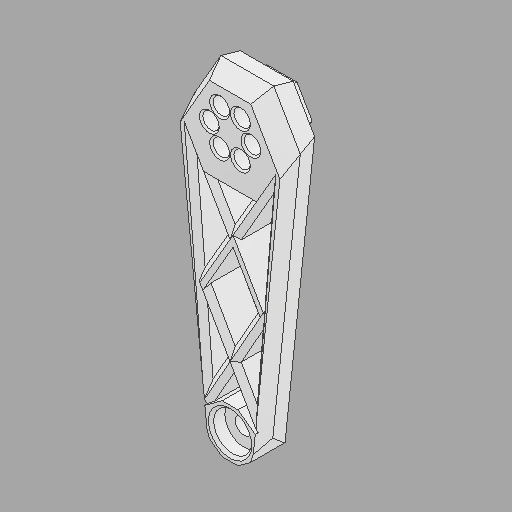
# Autodesk Inventor part: UPPER_LINKAGE_LH_V2
Saved by Autodesk Inventor 2025.2 (Build 292293000, 293)
## iProperties
Created: 2026-05-25
Part Number: UPPER_LINKAGE_LH_V2
Material: ABS Plastic
Document SubType Name: Modeling
Designer: Ben
Density: 1.06 g/cm^3
Appearance: Smooth - White
Mass: 110.874 g
Surface Area: 371.231 cm^2
Volume: 104.598 cm^3
Author: Ben
Autodesk Inventor part; units mm, degrees
ref_plane "YZ Plane" through (0, 0, 0) normal (1, 0, 0) x (0, 1, 0)
ref_plane "XZ Plane" through (0, 0, 0) normal (0, 1, 0) x (-1, 0, 0)
ref_plane "XY Plane" through (0, 0, 0) normal (0, 0, 1) x (1, 0, 0)
sketch "Sketch1" plane through (0, 0, 0) normal (0, 0, 1) x (1, 0, 0)
  circle A0 centre (0, 0) radius 26.5
  circle A1 centre (0, -150) radius 14
  line L0 (-26.407826, -2.208333) -> (-13.951304, -151.166667)
  line L1 (26.407826, -2.208333) -> (13.951304, -151.166667)
  line L2 (-42.83939, 0) -> (42.83939, 0)
  line L3 (30.599564, 0) -> (15.299782, 26.5)
  line L4 (15.299782, 26.5) -> (-15.299782, 26.5)
  line L5 (-15.299782, 26.5) -> (-30.599564, 0)
  line L6 (14.720471, -150) -> (11.909111, -158.652476)
  line L7 (11.909111, -158.652476) -> (4.548876, -164)
  line L8 (4.548876, -164) -> (-4.548876, -164)
  line L9 (-4.548876, -164) -> (-11.909111, -158.652476)
  line L10 (-11.909111, -158.652476) -> (-14.720471, -150)
  line L11 (30.599564, 0) -> (14.720471, -150)
  line L12 (-30.599564, 0) -> (-14.720471, -150)
  line L13 (30.599564, 0) -> (15.299782, -26.5)
  line L14 (15.299782, -26.5) -> (-15.299782, -26.5)
  line L15 (-30.599564, 0) -> (-15.299782, -26.5)
  line L16 (14.720471, -150) -> (11.909111, -141.347524)
  line L17 (11.909111, -141.347524) -> (4.548876, -136)
  line L18 (4.548876, -136) -> (-4.548876, -136)
  line L19 (-4.548876, -136) -> (-11.909111, -141.347524)
  line L20 (-11.909111, -141.347524) -> (-14.720471, -150)
  line L21 (22.949673, -13.25) -> (11.909111, -141.347524)
  line L22 (-11.909111, -141.347524) -> (-22.949673, -13.25)
  line L23 (22.341795, -20.302876) -> (-16.537733, -87.644193)
  line L24 (11.835681, -26.5) -> (-17.437654, -77.202903)
  line L25 (15.299782, -26.5) -> (-16.987693, -82.423548) construction
  line L26 (-15.299782, -26.5) -> (16.987693, -82.423548) construction
  line L27 (-22.341795, -20.302876) -> (16.537733, -87.644193)
  line L28 (17.437654, -77.202903) -> (-11.835681, -26.5)
  line L29 (17.437654, -77.202903) -> (-12.821294, -130.763976)
  line L30 (16.197037, -91.597102) -> (-11.909111, -141.347524)
  line L31 (-17.437654, -77.202903) -> (12.821294, -130.763976)
  line L32 (-16.197037, -91.597102) -> (11.909111, -141.347524)
  point P0 (-26.5, 0)
  point P1 (26.5, 0)
  point P2 (-22.949673, 13.25)
  point P3 (0, 26.5)
  point P4 (22.949673, 13.25)
  point P5 (13.314791, -154.326238)
  point P6 (-13.314791, -154.326238)
  point P7 (-8.228994, -161.326238)
  point P8 (0, -164)
  point P9 (8.228994, -161.326238)
  point P10 (-3.464102, -53)
  point P11 (0, -59)
  point P12 (3.464102, -53)
  point P13 (0, -47)
  point P14 (3.445641, -114.168224)
  point P15 (14.011179, -83.268074)
  point P16 (0, -108.069127)
  point P17 (-14.011179, -83.268074)
  point P18 (-3.445641, -114.168224)
  point P19 (0, -120.267321)
  dimension "d0" = 53
  dimension "d1" = 28
  dimension "d2" = 150
  dimension "d50" = 360
  dimension "d60" = 360
  dimension "d68" = 6
  dimension "d69" = 6
  dimension "d70" = 6
  dimension "d71" = 6
  constraints: 60 end point, 6 tangent, 5 parallel, 4 point on circle, 3 coincident, 3 point on line, 2 centre point, 2 collinear, 2 horizontal, 2 midpoint, 1 horizontal alignment, 1 vertical alignment, 40 other
  measures "d0" diameter of A0
  measures "d1" diameter of A1
  measures "d2" distance of A1.centre point (0, 0)
  measures "d68" distance between parallel lines of L24 L23
  measures "d69" distance between parallel lines of L27 L28
  measures "d70" distance between parallel lines of L32 L31
  measures "d71" distance between parallel lines of L30 L29
extrude "Extrusion1" add sketch "Sketch1" along normal blind 20 contours A0 L2 | L0 L15 L2 A0 | A0 L15 L0 | A0 L14 L15 | L22 L20 L0 L15 | L15 L14 L28 L24 L27 L22 | L2 L5 A0 | A0 L2 | L0 L20 L12 L15 | A0 L13 L14 | L5 L4 A0 | L2 L13 L1 A0 | A0 L3 L2 | L20 A1 L0 | L0 A1 L10 L20 | L21 L23 L28 L24 L14 L13 | A0 L1 L13 | L13 L1 L16 L21 | L31 L23 L22 | L24 L27 L23 L31 | L24 L28 L23 L27 | L4 L3 A0 | L11 L16 L1 L13 | A1 | L20 L19 A1 | L23 L31 L29 L32 L22 | L23 L28 L29 L27 | A1 L9 L10 | L6 A1 L1 L16 | L19 L18 A1 | L22 L29 L32 L30 | L1 A1 L16 | L21 L27 L29 | L31 L30 L32 L29 | L29 L27 L21 L30 L31 | A1 L8 L9 | L6 L7 A1 | L18 L17 A1 | L30 L31 L21 L32 | A1 L17 L16 | A1 L7 L8
sketch "Sketch2" plane through (0, 0, 20) normal (0, 0, 1) x (1, 0, 0)
  line L0 (0, -202.1) -> (0, 64.6)
  line L1 (-6, 10.392305) -> (0, 0) construction
  point P0 (6, 10.392305)
  point P1 (-6, -10.392305)
  point P2 (-12, 0)
  point P3 (12, 0)
  point P4 (6, -10.392305)
  dimension "d18" = 12
  dimension "d19" = 12
  dimension "d22" = 360
  constraints: 2 coincident, 2 end point, 1 symmetric about line, 8 other
  measures "d18" distance of point (6, 10.392) L1.start
  measures "d19" distance of L1.start L1.end
sketch "Sketch3" plane through (0, 0, 20) normal (0, 0, 1) x (1, 0, 0)
  arc A0 (-14.98591, -150.65) -> (14.98591, -150.65) centre (0, -150) ccw
  point P0 (0, 0)
  constraints: 1 coincident
hole "Hole2" at (0, -150, 20) direction (0, 0, -1) diameter 10 end through all counterbore diameter 22 counterbore depth 8
chamfer "Chamfer4" distance 1.5 angle 45 1 edges at (0, -139, 20)
chamfer "Chamfer5" distance 10 angle 30 1 edges at (22.9497, 13.25, 20) measured on face at (22.9497, 13.25, 19.5)
chamfer "Chamfer6" distance 10 angle 30 1 edges at (-3.3333, 26.5, 20) measured on face at (-3.3333, 26.5, 19.5)
chamfer "Chamfer7" distance 10 angle 30 1 edges at (-24.6163, 10.3632, 20) measured on face at (-24.6163, 10.3632, 19.5)
chamfer "Chamfer8" distance 10 angle 5 1 edges at (-22.1435, -79.8789, 20) measured on face at (-22.1435, -79.8789, 19.5)
chamfer "Chamfer9" distance 10 angle 5 1 edges at (22.1435, -79.8789, 20) measured on face at (22.1435, -79.8789, 19.5)
chamfer "Chamfer10" distance 3 angle 45 18 edges at (19.8897, -48.7529, 20) (12.9029, -36.6514, 20) (5.9178, -36.75, 20) (-5.9178, -36.75, 20) (-12.9029, -36.6514, 20) (-10.4509, -65.1015, 20) (-19.8897, -48.7529, 20) (7.0056, -71.134, 20) (-7.0056, -95.6686, 20) (-9.8213, -102.8827, 20) (-8.1335, -122.4661, 20) (-5.9546, -130.8074, 20) (5.9546, -130.8074, 20) (8.1335, -122.4661, 20) (14.5092, -111.1805, 20) (9.8213, -102.8827, 20) (7.0056, -95.6686, 20) (-14.5092, -111.1805, 20)
sketch "Sketch4" plane through (0, 0, 0) normal (0, 0, -1) x (-1, 0, 0)
  line L0 (-8.75, 15.155445) -> (-17.5, 0)
  line L1 (-17.5, 0) -> (-8.75, -15.155445)
  line L2 (-8.75, -15.155445) -> (8.75, -15.155445)
  line L3 (8.75, -15.155445) -> (17.5, 0)
  line L4 (17.5, 0) -> (8.75, 15.155445)
  line L5 (8.75, 15.155445) -> (-8.75, 15.155445)
  point P0 (0, 0)
  dimension "d91" = 17.5
  dimension "d94" = 360
  constraints: 12 end point, 3 parallel, 1 horizontal, 1 horizontal alignment, 7 other
  measures "d91" distance of point (0, 0) L0.end
extrude "Extrusion2" add sketch "Sketch4" along normal blind 10
hole "Hole3" at (-6, 10.392305, 20) at (6, 10.392305, 20) at (-6, -10.392305, 20) at (-12, 0, 20) at (12, 0, 20) at (6, -10.392305, 20) direction (0, 0, -1) diameter 4.5 end through all counterbore diameter 9.5 counterbore depth 15
chamfer "Chamfer11" distance 1 angle 45 6 edges at (-12, 4.75, 20) (-6, -5.6423, 20) (6, -5.6423, 20) (12, 4.75, 20) (6, 15.1423, 20) (-6, 15.1423, 20)
chamfer "Chamfer12" distance 2 distance2 10 6 edges at (0, 15.1554, 0) (13.125, 7.5777, 0) (13.125, -7.5777, 0) (0, -15.1554, 0) (-13.125, -7.5777, 0) (-13.125, 7.5777, 0) measured on face at (13.558, -7.8277, 0) measured on face at (0, 15.6554, 0) measured on face at (13.558, 7.8277, 0) measured on face at (-13.558, 7.8277, 0) measured on face at (0, -15.6554, 0) measured on face at (-13.558, -7.8277, 0)
chamfer "Chamfer13" distance 10 distance2 2 1 edges at (0, 26.5, 0) measured on face at (0, 26.5, 0.5)
chamfer "Chamfer14" distance 10 distance2 2 1 edges at (-23.527, 12.2501, 0) measured on face at (-23.527, 12.2501, 0.5)
chamfer "Chamfer15" distance 10 distance2 2 1 edges at (-22.4811, -76.69, 0) measured on face at (-22.4811, -76.69, 0.5)
chamfer "Chamfer16" distance 10 distance2 2 1 edges at (22.66, -75, 0) measured on face at (22.66, -75, 0.5)
body "Solid1"
